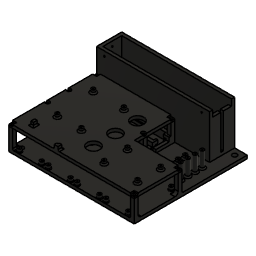
electronics_baseplate (Autodesk Fusion 360 design; units mm, degrees)
Autodesk Fusion 360 part; units mm, degrees
(part 1 of 2)
sketch "Sketch1" plane through (0, 0, 0) normal (0, 1, 0) x (1, 0, 0)
  line L0 (0, 0) -> (200, 0)
  line L1 (200, 0) -> (200, 180)
  line L2 (200, 180) -> (0, 180)
  line L3 (0, 180) -> (0, 0)
  dimension "d3_1" = 200
  dimension "d4_1" = 180
  constraint horizontal L0
  constraint vertical L1
  constraint horizontal L2
  constraint vertical L3
  constraint coincident L0.start L3.end
  measures "d3_1" distance of L0.start L0.end
  measures "d4_1" distance of L0.start L2.end
extrude "Extrude1" add sketch "Sketch1" along normal blind 5 makes body 1
sketch "Sketch3" plane through (0, 0, 0) normal (0, -1, 0) x (1, 0, 0)
  line L0 (0, 0) -> (0, -180)
  line L1 (0, -180) -> (200, -180)
  line L2 (200, -180) -> (200, 0)
  line L3 (200, 0) -> (0, 0)
  line L4 (10, -170) -> (190, -170)
  line L5 (190, -170) -> (190, -10)
  line L6 (190, -10) -> (10, -10)
  line L7 (10, -10) -> (10, -170)
  circle A0 centre (10, -10) radius 2
  circle A1 centre (190, -10) radius 2
  circle A2 centre (10, -170) radius 2
  circle A3 centre (190, -170) radius 2
  dimension "d13_1" = 4
  dimension "d14_1" = 4
  dimension "d15_2" = 4
  dimension "d16" = 4
  constraint coincident L6.end L7.start
  constraint coincident L5.end L6.start
  constraint coincident L4.start L7.end
  constraint coincident L4.end L5.start
  measures "d13_1" diameter of A0
  measures "d14_1" diameter of A1
  measures "d15_2" diameter of A2
  measures "d16" diameter of A3
extrude "Extrude2" cut sketch "Sketch3" against normal up to surface (5 mm away) contours L4 L7 A2 | L4 L7 A2 | L4 L5 A3 | L4 L5 A3 | L6 L7 A0 | L6 L7 A0 | L5 L6 A1 | L5 L6 A1 bodies 1
chamfer "Chamfer1" distance 1.75 distance2 5 4 edges at (8.1353, 5, -170.7232) (188.1353, 5, -170.7232) (8.1353, 5, -10.7232) (188.1353, 5, -10.7232) measured on face at (70.4714, 5, -116.1953) measured on face at (70.4714, 5, -116.1953) measured on face at (70.4714, 5, -116.1953) measured on face at (70.4714, 5, -116.1953) on bodies 1
sketch "Sketch4" plane through (0, 5, 0) normal (0, 1, 0) x (-1, 0, 0)
  circle A0 centre (-10, -10) radius 3.75
  circle A1 centre (-10, -170) radius 3.75
  line L0 (0, -180) -> (0, 0)
  line L1 (0, 0) -> (-200, 0)
  line L2 (-200, 0) -> (-200, -180)
  line L3 (-200, -180) -> (0, -180)
  circle A2 centre (-190, -170) radius 3.75
  circle A3 centre (-190, -10) radius 3.75
  line L4 (0, -180) -> (-180, -180)
  line L5 (-180, -180) -> (-180, -140)
  line L6 (-180, -140) -> (0, -140)
  line L7 (0, -140) -> (0, -180)
  line L8 (-5, -175) -> (-175, -175)
  line L9 (-175, -175) -> (-175, -145)
  line L10 (-175, -145) -> (-5, -145)
  line L11 (-5, -145) -> (-5, -175)
  dimension "d25_1" = 180
  dimension "d26_2" = 40
  dimension "d27_2" = 5
  constraint horizontal L4
  constraint vertical L5
  constraint horizontal L6
  constraint vertical L7
  constraint coincident L0.start L3.end
  measures "d25_1" distance of L0.start L4.end
  measures "d26_2" distance of L0.start L6.end
extrude "Extrude3" add sketch "Sketch4" along normal blind 70 contours L0 L3 L4 L5 L6 L7 bodies 1
sketch "Sketch5" plane through (0, 75, 0) normal (0, 1, 0) x (-1, 0, 0)
  line L0 (-175, -145) -> (-5, -145)
  line L1 (-5, -145) -> (-5, -175)
  line L2 (-5, -175) -> (-175, -175)
  line L3 (-175, -175) -> (-175, -145)
  line L4 (0, -140) -> (-180, -140)
  line L5 (-180, -140) -> (-180, -180)
  line L6 (-180, -180) -> (0, -180)
  line L7 (0, -180) -> (0, -140)
  line L8 (-180, -180) -> (-175, -180)
  line L9 (-175, -180) -> (-175, -175)
  line L10 (-175, -175) -> (-180, -175)
  line L11 (-180, -175) -> (-180, -180)
  line L12 (-175, -145) -> (-180, -145)
  line L13 (-180, -145) -> (-180, -140)
  line L14 (-180, -140) -> (-175, -140)
  line L15 (-175, -140) -> (-175, -145)
  constraint horizontal L8
  constraint vertical L9
  constraint horizontal L10
  constraint vertical L11
  constraint coincident L2.end L3.start
  constraint coincident L5.end L6.start
  constraint horizontal L12
  constraint vertical L13
  constraint horizontal L14
  constraint vertical L15
  constraint coincident L4.end L5.start
  constraint coincident L0.start L3.end
extrude "Extrude4" cut sketch "Sketch5" against normal blind 10 contours L3 L5 L10 L12 bodies 1
sketch "Sketch6" plane through (0, 65, 0) normal (0, 1, 0) x (-1, 0, 0)
  line L0 (-175, -175) -> (-175, -145)
  line L1 (-175, -145) -> (-180, -145)
  line L2 (-180, -145) -> (-180, -175)
  line L3 (-180, -175) -> (-175, -175)
  line L4 (-175, -160) -> (-180, -160)
  line L5 (-180, -162) -> (-175, -162)
  line L6 (-175, -162) -> (-175, -158)
  line L7 (-175, -158) -> (-180, -158)
  line L8 (-180, -158) -> (-180, -162)
  line L9 (-180, -162) -> (-175, -158) construction
  line L10 (-175, -162) -> (-180, -158) construction
  point P0 (-177.5, -160)
  dimension "d34_2" = 5
  dimension "d35_2" = 4
  constraint midpoint L0 L4.start
  constraint midpoint L2 L4.end
  constraint horizontal L5
  constraint perpendicular L5 L6
  constraint parallel L5 L7
  constraint parallel L6 L8
  constraint coincident L9 P0
  constraint coincident L10 P0
  constraint midpoint L4 P0
  measures "d34_2" distance of L6.end L7.end
  measures "d35_2" distance of L5.end L6.end
extrude "Extrude5" cut sketch "Sketch6" against normal blind 55 contours L0 L2 L4 L5 L6 L8 | L0 L2 L4 L6 L7 L8 bodies 1
sketch "Sketch7" plane through (0, 5, 0) normal (0, 1, 0) x (-1, 0, 0)
  circle A0 centre (-190, -10) radius 3.75
  circle A1 centre (-190, -170) radius 3.75
  line L0 (-180, -180) -> (-180, -140)
  line L1 (-180, -140) -> (0, -140)
  line L2 (0, -140) -> (0, 0)
  line L3 (0, 0) -> (-200, 0)
  line L4 (-200, 0) -> (-200, -180)
  line L5 (-200, -180) -> (-180, -180)
  circle A2 centre (-10, -10) radius 3.75
  line L6 (-100, 0) -> (-100, -140)
  line L7 (-100, 0) -> (-98.5, 0)
  line L8 (-98.5, 0) -> (-98.5, -76)
  line L9 (-98.5, -76) -> (-100, -76)
  line L10 (-100, -76) -> (-100, 0)
  line L11 (-98.5, 0) -> (-55.5, 0)
  line L12 (-55.5, 0) -> (-55.5, -76)
  line L13 (-55.5, -76) -> (-98.5, -76)
  line L14 (-98.5, -76) -> (-98.5, 0)
  line L15 (-55.5, 0) -> (-52.5, 0)
  line L16 (-52.5, 0) -> (-52.5, -76)
  line L17 (-52.5, -76) -> (-55.5, -76)
  line L18 (-55.5, -76) -> (-55.5, 0)
  line L19 (-52.5, 0) -> (-9.5, 0)
  line L20 (-9.5, 0) -> (-9.5, -76)
  line L21 (-9.5, -76) -> (-52.5, -76)
  line L22 (-52.5, -76) -> (-52.5, 0)
  line L23 (-48.75, -3.75) -> (-13.25, -3.75)
  line L24 (-13.25, -3.75) -> (-13.25, -72.25)
  line L25 (-13.25, -72.25) -> (-48.75, -72.25)
  line L26 (-48.75, -72.25) -> (-48.75, -3.75)
  line L27 (-59.25, -3.75) -> (-59.25, -72.25)
  line L28 (-59.25, -72.25) -> (-94.75, -72.25)
  line L29 (-94.75, -72.25) -> (-94.75, -3.75)
  line L30 (-94.75, -3.75) -> (-59.25, -3.75)
  circle A3 centre (-13.25, -3.75) radius 3
  circle A4 centre (-13.25, -72.25) radius 3
  circle A5 centre (-48.75, -72.25) radius 3
  circle A6 centre (-59.25, -72.25) radius 3
  circle A7 centre (-94.75, -72.25) radius 3
  circle A8 centre (-59.25, -3.75) radius 3
  circle A9 centre (-94.75, -3.75) radius 3
  line L31 (-100, -76) -> (-100, 0)
  line L32 (-101.5, -76) -> (-101.5, 0)
  line L33 (-147.5, -76) -> (-144.5, -76)
  circle A10 centre (-140.75, -3.75) radius 3
  line L34 (-101.5, 0) -> (-101.5, -76)
  line L35 (-147.5, 0) -> (-147.5, -76)
  line L36 (-190.5, 0) -> (-190.5, -76)
  line L37 (-144.5, 0) -> (-147.5, 0)
  line L38 (-147.5, -76) -> (-147.5, 0)
  line L39 (-144.5, 0) -> (-144.5, -76)
  line L40 (-140.75, -72.25) -> (-105.25, -72.25)
  line L41 (-105.25, -72.25) -> (-105.25, -3.75)
  line L42 (-140.75, -3.75) -> (-140.75, -72.25)
  line L43 (-101.5, 0) -> (-144.5, 0)
  line L44 (-147.5, 0) -> (-190.5, 0)
  circle A11 centre (-186.75, -72.25) radius 3
  circle A12 centre (-151.25, -72.25) radius 3
  line L45 (-151.25, -72.25) -> (-151.25, -3.75)
  circle A13 centre (-186.75, -3.75) radius 3
  line L46 (-101.5, -76) -> (-100, -76)
  line L47 (-144.5, -76) -> (-101.5, -76)
  line L48 (-100, 0) -> (-101.5, 0)
  line L49 (-105.25, -3.75) -> (-140.75, -3.75)
  circle A14 centre (-105.25, -3.75) radius 3
  circle A15 centre (-105.25, -72.25) radius 3
  line L50 (-144.5, -76) -> (-144.5, 0)
  line L51 (-186.75, -72.25) -> (-151.25, -72.25)
  circle A16 centre (-140.75, -72.25) radius 3
  line L52 (-186.75, -3.75) -> (-186.75, -72.25)
  line L53 (-190.5, -76) -> (-147.5, -76)
  line L54 (-151.25, -3.75) -> (-186.75, -3.75)
  circle A17 centre (-48.75, -3.75) radius 3
  circle A18 centre (-151.25, -3.75) radius 3
  point P0 (-190, -10)
  dimension "d46_2" = 1.5
  dimension "d47_2" = 76
  dimension "d48_2" = 43
  dimension "d49_2" = 76
  dimension "d50_2" = 3
  dimension "d51_2" = 76
  dimension "d52_2" = 43
  dimension "d53_2" = 76
  dimension "d54_2" = 3.75
  dimension "d55_2" = 3.75
  dimension "d56_2" = 6
  dimension "d57_2" = 6
  dimension "d58_2" = 6
  dimension "d59_2" = 6
  dimension "d60_2" = 6
  dimension "d61_2" = 6
  dimension "d62_2" = 6
  dimension "d63_2" = 6
  constraint midpoint L3 L6.start
  constraint coincident L1 L6.end
  constraint perpendicular L1 L6
  constraint horizontal L7
  constraint vertical L8
  constraint horizontal L9
  constraint vertical L10
  constraint horizontal L11
  constraint vertical L12
  constraint horizontal L13
  constraint vertical L14
  constraint horizontal L15
  constraint vertical L16
  constraint horizontal L17
  constraint vertical L18
  constraint horizontal L19
  constraint vertical L20
  constraint horizontal L21
  constraint vertical L22
  constraint coincident L23.end L24.start
  constraint coincident L24.end L25.start
  constraint coincident L25.end L26.start
  constraint coincident L27.end L28.start
  constraint coincident L28.end L29.start
  constraint coincident L27.start L30.end
  constraint coincident L29.end L30.start
  constraint symmetric A2.centre L6 P0
  constraint symmetric L7.start L6 L10.end
  constraint symmetric L6 L7.end L32.end
  constraint symmetric L6 L8.end L32.start
  constraint symmetric L6 L9.end L10.start
  constraint symmetric L6 L11.end L37.start
  constraint symmetric L6 L12.end L33.end
  constraint symmetric L6 L15.end L35.start
  constraint symmetric L6 L16.end L33.start
  constraint symmetric L6 L19.end L36.start
  constraint symmetric L6 L20.end L36.end
  constraint symmetric L6 L23.start L45.end
  constraint symmetric L6 L23.end A13.centre
  constraint symmetric L6 L24.end A11.centre
  constraint symmetric L6 L25.end A12.centre
  constraint symmetric L6 L27.start A10.centre
  constraint symmetric L6 L27.end L40.start
  constraint symmetric L6 L28.end L40.end
  constraint symmetric L6 L29.end L41.end
  constraint symmetric L6 A3 A13
  constraint symmetric L6 A4 A11
  constraint symmetric L6 A5 A12
  constraint symmetric L6 A6 A16
  constraint symmetric L6 A7 A15
  constraint symmetric L6 A8 A10
  constraint symmetric L6 A9 A14
  constraint coincident L23.start L26.end
  constraint symmetric L6 A17 A18
  measures "d46_2" distance of L6.start L7.end
  measures "d47_2" distance of L6.start L9.end
  measures "d48_2" distance of L7.end L11.end
  measures "d49_2" distance of L7.end L8.end
  measures "d50_2" distance of L11.end L15.end
  measures "d51_2" distance of L11.end L12.end
  measures "d52_2" distance of L15.end L19.end
  measures "d53_2" distance of L15.end L16.end
  measures "d56_2" diameter of A3
  measures "d57_2" diameter of A4
  measures "d58_2" diameter of A5
  measures "d59_2" diameter of A6
  measures "d60_2" diameter of A7
  measures "d61_2" diameter of A8
  measures "d62_2" diameter of A9
  measures "d63_2" diameter of A17
extrude "Extrude6" add sketch "Sketch7" along normal blind 5 contours A13 L52 L54 | A13 L52 L54 | A11 L51 L52 | A11 L51 L52 | L45 L54 A18 | L45 L54 A18 | A12 L45 L51 | A12 L45 L51 | L23 L24 A3 | L23 L24 A3 | L24 L25 A4 | L24 L25 A4 | L23 L26 A17 | L23 L26 A17 | L25 L26 A5 | L25 L26 A5 | L27 L30 A8 | L27 L30 A8 | L27 L28 A6 | L27 L28 A6 | L29 L30 A9 | L29 L30 A9 | L28 L29 A7 | L28 L29 A7 | A10 L42 L49 | A10 L42 L49 | L41 L49 A14 | L41 L49 A14 | L40 L42 A16 | L40 L42 A16 | L40 L41 A15 | L40 L41 A15 bodies 1
fillet "Fillet1" radius 1 16 edges at (16.047, 5, -71.1652) (51.547, 5, -71.1652) (62.047, 5, -71.1652) (16.047, 5, -2.6652) (51.547, 5, -2.6652) (62.047, 5, -2.6652) (97.547, 5, -71.1652) (108.047, 5, -71.1652) (97.547, 5, -2.6652) (108.047, 5, -2.6652) (143.547, 5, -71.1652) (154.047, 5, -71.1652) (143.547, 5, -2.6652) (154.047, 5, -2.6652) (189.547, 5, -71.1652) (189.547, 5, -2.6652) on bodies 1
sketch "Sketch8" plane through (0, 5, 0) normal (0, 1, 0) x (-1, 0, 0)
  arc A0 (-188.1419, 0) -> (-189.8707, -6.2522) centre (-186.75, -3.75) ccw
  line L0 (-188.1419, 0) -> (-200, 0)
  line L1 (-200, 0) -> (-200, -180)
  line L2 (-200, -180) -> (-180, -180)
  line L3 (-180, -180) -> (-180, -140)
  line L4 (-180, -140) -> (0, -140)
  line L5 (0, -140) -> (0, 0)
  line L6 (0, 0) -> (-11.8581, 0)
  arc A1 (-10.1293, -6.2522) -> (-11.8581, 0) centre (-13.25, -3.75) ccw
  arc A2 (-12.9938, -7.7418) -> (-10.1293, -6.2522) centre (-10, -10) ccw
  arc A3 (-14.6419, 0) -> (-12.9938, -7.7418) centre (-13.25, -3.75) ccw
  line L7 (-14.6419, 0) -> (-47.3581, 0)
  arc A4 (-50.1419, 0) -> (-47.3581, 0) centre (-48.75, -3.75) ccw
  line L8 (-50.1419, 0) -> (-57.8581, 0)
  arc A5 (-60.6419, 0) -> (-57.8581, 0) centre (-59.25, -3.75) ccw
  line L9 (-60.6419, 0) -> (-93.3581, 0)
  arc A6 (-96.1419, 0) -> (-93.3581, 0) centre (-94.75, -3.75) ccw
  line L10 (-96.1419, 0) -> (-103.8581, 0)
  arc A7 (-106.6419, 0) -> (-103.8581, 0) centre (-105.25, -3.75) ccw
  line L11 (-106.6419, 0) -> (-139.3581, 0)
  arc A8 (-142.1419, 0) -> (-139.3581, 0) centre (-140.75, -3.75) ccw
  line L12 (-142.1419, 0) -> (-149.8581, 0)
  arc A9 (-152.6419, 0) -> (-149.8581, 0) centre (-151.25, -3.75) ccw
  line L13 (-152.6419, 0) -> (-185.3581, 0)
  arc A10 (-187.0062, -7.7418) -> (-185.3581, 0) centre (-186.75, -3.75) ccw
  arc A11 (-189.8707, -6.2522) -> (-187.0062, -7.7418) centre (-190, -10) ccw
  circle A12 centre (-151.25, -72.25) radius 4
  circle A13 centre (-105.25, -72.25) radius 4
  circle A14 centre (-59.25, -72.25) radius 4
  circle A15 centre (-13.25, -72.25) radius 4
  circle A16 centre (-190, -170) radius 3.75
  circle A17 centre (-48.75, -72.25) radius 4
  circle A18 centre (-94.75, -72.25) radius 4
  circle A19 centre (-140.75, -72.25) radius 4
  circle A20 centre (-186.75, -72.25) radius 4
  line L14 (0, -140) -> (-55.5, -140)
  line L15 (-55.5, -140) -> (-55.5, -110)
  line L16 (-55.5, -110) -> (0, -110)
  line L17 (0, -110) -> (0, -140)
  line L18 (-55.5, -140) -> (-124.5, -140)
  line L19 (-124.5, -140) -> (-124.5, -110)
  line L20 (-124.5, -110) -> (-55.5, -110)
  line L21 (-55.5, -110) -> (-55.5, -140)
  line L22 (-60.5, -135) -> (-119.5, -135)
  line L23 (-119.5, -135) -> (-119.5, -115)
  line L24 (-119.5, -115) -> (-60.5, -115)
  line L25 (-60.5, -115) -> (-60.5, -135)
  line L26 (-60.5, -135) -> (-61.5, -135)
  line L27 (-61.5, -135) -> (-61.5, -115)
  line L28 (-61.5, -115) -> (-60.5, -115)
  line L29 (-60.5, -115) -> (-60.5, -135)
  line L30 (-60.5, -135) -> (-85.5, -135)
  line L31 (-85.5, -135) -> (-85.5, -134)
  line L32 (-85.5, -134) -> (-60.5, -134)
  line L33 (-60.5, -134) -> (-60.5, -135)
  line L34 (-119.5, -135) -> (-115.5, -135)
  line L35 (-115.5, -135) -> (-115.5, -131)
  line L36 (-115.5, -131) -> (-119.5, -131)
  line L37 (-119.5, -131) -> (-119.5, -135)
  line L38 (-119.5, -115) -> (-115.5, -115)
  line L39 (-115.5, -115) -> (-115.5, -119)
  line L40 (-115.5, -119) -> (-119.5, -119)
  line L41 (-119.5, -119) -> (-119.5, -115)
  line L42 (-119.5, -115) -> (-119.5, -110)
  line L43 (-119.5, -119) -> (-124.5, -119)
  line L44 (-119.5, -131) -> (-124.5, -131)
  line L45 (-60.5, -115) -> (-60.5, -110)
  dimension "d78_1" = 55.5
  dimension "d79_1" = 30
  dimension "d81_1" = 69
  dimension "d82_1" = 30
  dimension "d83_1" = 5
  dimension "d84_1" = 1
  dimension "d85_1" = 25
  dimension "d86_1" = 1
  dimension "d87_1" = 4
  dimension "d88_1" = 4
  dimension "d89_2" = 4
  dimension "d90_2" = 4
  constraint horizontal L14
  constraint vertical L15
  constraint horizontal L16
  constraint vertical L17
  constraint coincident L4.end L5.start
  constraint horizontal L18
  constraint vertical L19
  constraint horizontal L20
  constraint vertical L21
  constraint horizontal L26
  constraint vertical L27
  constraint horizontal L28
  constraint vertical L29
  constraint horizontal L30
  constraint vertical L31
  constraint horizontal L32
  constraint vertical L33
  constraint collinear L24 L28
  constraint horizontal L34
  constraint vertical L35
  constraint horizontal L36
  constraint vertical L37
  constraint horizontal L38
  constraint vertical L39
  constraint horizontal L40
  constraint vertical L41
  constraint coincident L20 L42.end
  constraint perpendicular L20 L42
  constraint coincident L19 L43.end
  constraint perpendicular L19 L43
  constraint coincident L19 L44.end
  constraint perpendicular L19 L44
  constraint coincident L20 L45.end
  constraint perpendicular L20 L45
  measures "d78_1" distance of L4.end L14.end
  measures "d79_1" distance of L4.end L16.end
  measures "d81_1" distance of L14.end L18.end
  measures "d82_1" distance of L14.end L15.end
  measures "d84_1" distance of L22.start L26.end
  measures "d85_1" distance of L22.start L30.end
  measures "d86_1" distance of L22.start L32.end
  measures "d87_1" distance of L22.end L34.end
  measures "d88_1" distance of L22.end L36.end
  measures "d89_2" distance of L23.end L38.end
  measures "d90_2" distance of L23.end L40.end
extrude "Extrude7" add sketch "Sketch8" along normal blind 11.5 contours L4 L15 L18 L19 L20 L21 L22 L23 L25 L26 L29 L30 L33 L34 L37 L44 L45 | L19 L20 L23 L41 L42 L43 | L22 L23 L34 L35 L36 L37 | L24 L25 L27 L28 L29 L32 | L22 L25 L26 L27 L29 L30 L32 L33 | L22 L27 L30 L31 L32 bodies 1
extrude "Extrude8" add sketch "Sketch8" along normal blind 5 contours L19 L23 L43 L44 | L20 L24 L28 L38 L42 L45 | L23 L24 L38 L39 L40 L41 bodies 1
sketch "Sketch9" plane through (0, 0, -110) normal (0, 0, 1) x (1, 0, 0)
  line L0 (55.5, 5) -> (124.5, 5)
  line L1 (124.5, 5) -> (124.5, 16.5)
  line L2 (124.5, 16.5) -> (119.5, 16.5)
  line L3 (119.5, 16.5) -> (119.5, 10)
  line L4 (119.5, 10) -> (60.5, 10)
  line L5 (60.5, 10) -> (60.5, 16.5)
  line L6 (60.5, 16.5) -> (55.5, 16.5)
  line L7 (55.5, 16.5) -> (55.5, 5)
  line L8 (60.5, 10) -> (119.5, 10)
  line L9 (119.5, 10) -> (119.5, 12)
  line L10 (119.5, 12) -> (60.5, 12)
  line L11 (60.5, 12) -> (60.5, 10)
  dimension "d95_1" = 2
  constraint horizontal L8
  constraint vertical L9
  constraint horizontal L10
  constraint vertical L11
  constraint coincident L3 L9.end
  constraint coincident L4.end L5.start
  measures "d95_1" distance of L4.end L10.end
extrude "Extrude9" cut sketch "Sketch9" against normal up to surface (25 mm away) contours L3 L4 L5 L8 L9 L10 L11 bodies 1
sketch "Sketch14" plane through (0, 0, -110) normal (0, 0, 1) x (1, 0, 0)
  line L0 (55.5, 5) -> (124.5, 5)
  line L1 (124.5, 5) -> (124.5, 16.5)
  line L2 (124.5, 16.5) -> (119.5, 16.5)
  line L3 (119.5, 16.5) -> (119.5, 10)
  line L4 (119.5, 10) -> (60.5, 10)
  line L5 (60.5, 10) -> (60.5, 16.5)
  line L6 (60.5, 16.5) -> (55.5, 16.5)
  line L7 (55.5, 16.5) -> (55.5, 5)
  line L8 (60.5, 5) -> (119.5, 5)
  line L9 (119.5, 5) -> (119.5, 10)
  line L10 (119.5, 10) -> (60.5, 10)
  line L11 (60.5, 10) -> (60.5, 5)
  line L12 (60.5, 10) -> (64.5, 10)
  line L13 (64.5, 10) -> (64.5, 5)
  line L14 (64.5, 5) -> (60.5, 5)
  line L15 (60.5, 5) -> (60.5, 10)
  line L16 (119.5, 10) -> (115.5, 10)
  line L17 (115.5, 10) -> (115.5, 5)
  line L18 (115.5, 5) -> (119.5, 5)
  line L19 (119.5, 5) -> (119.5, 10)
  line L20 (64.5, 10) -> (68.5, 10)
  line L21 (68.5, 10) -> (68.5, 7)
  line L22 (68.5, 7) -> (64.5, 7)
  line L23 (64.5, 7) -> (64.5, 10)
  line L24 (115.5, 10) -> (111.5, 10)
  line L25 (111.5, 10) -> (111.5, 7)
  line L26 (111.5, 7) -> (115.5, 7)
  line L27 (115.5, 7) -> (115.5, 10)
  line L28 (68.5, 7) -> (111.5, 7)
  line L29 (90, 10) -> (90, 7)
  line L30 (115.5, 7) -> (119.5, 7)
  line L31 (88, 10) -> (92, 10)
  line L32 (92, 10) -> (92, 7)
  line L33 (92, 7) -> (88, 7)
  line L34 (88, 7) -> (88, 10)
  line L35 (88, 10) -> (92, 7) construction
  line L36 (92, 10) -> (88, 7) construction
  point P0 (90, 8.5)
  dimension "d106_1" = 4
  dimension "d107_1" = 4
  dimension "d108_1" = 4
  dimension "d109" = 3
  dimension "d110" = 4
  dimension "d111_1" = 3
  dimension "d112_1" = 4
  constraint horizontal L8
  constraint vertical L9
  constraint horizontal L10
  constraint vertical L11
  constraint coincident L3.end L4.start
  constraint coincident L0 L8.start
  constraint collinear L5 L11
  constraint horizontal L12
  constraint vertical L13
  constraint horizontal L14
  constraint vertical L15
  constraint horizontal L16
  constraint vertical L17
  constraint horizontal L18
  constraint vertical L19
  constraint collinear L8 L14
  constraint collinear L8 L18
  constraint horizontal L20
  constraint vertical L21
  constraint horizontal L22
  constraint vertical L23
  constraint horizontal L24
  constraint vertical L25
  constraint horizontal L26
  constraint vertical L27
  constraint midpoint L10 L29.start
  constraint midpoint L28 L29.end
  constraint coincident L9 L30.end
  constraint perpendicular L9 L30
  constraint horizontal L31
  constraint perpendicular L31 L32
  constraint parallel L31 L33
  constraint parallel L32 L34
  constraint coincident L35 P0
  constraint coincident L36 P0
  constraint midpoint L29 P0
  constraint collinear L10 L31
  measures "d106_1" distance of L4.end L12.end
  measures "d107_1" distance of L3.end L16.end
  measures "d108_1" distance of L12.end L20.end
  measures "d109" distance of L12.end L22.end
  measures "d110" distance of L16.end L24.end
  measures "d111_1" distance of L16.end L26.end
  measures "d112_1" distance of L32.end L33.end
extrude "Extrude11" cut sketch "Sketch14" against normal up to surface (5 mm away) contours L4 L10 L13 L20 L21 L22 L23 | L4 L10 L17 L24 L25 L26 L27 | L4 L10 L28 L29 L31 L33 L34 | L4 L10 L28 L29 L31 L32 L33 bodies 1
extrude "Extrude12" cut sketch "Sketch14" against normal up to surface (9 mm away) contours L4 L9 L10 L16 L17 L19 L27 L30 bodies 1
sketch "Sketch15" plane through (0, 5, 0) normal (0, 1, 0) x (-1, 0, 0)
  line L0 (-124.5, -110) -> (-55.5, -110)
  line L1 (-55.5, -110) -> (-55.5, -140)
  line L2 (-55.5, -140) -> (0, -140)
  line L3 (0, -140) -> (0, 0)
  line L4 (0, 0) -> (-11.8581, 0)
  arc A0 (-10.1293, -6.2522) -> (-11.8581, 0) centre (-13.25, -3.75) ccw
  arc A1 (-12.9938, -7.7418) -> (-10.1293, -6.2522) centre (-10, -10) ccw
  arc A2 (-14.6419, 0) -> (-12.9938, -7.7418) centre (-13.25, -3.75) ccw
  line L5 (-14.6419, 0) -> (-47.3581, 0)
  arc A3 (-50.1419, 0) -> (-47.3581, 0) centre (-48.75, -3.75) ccw
  line L6 (-50.1419, 0) -> (-57.8581, 0)
  arc A4 (-60.6419, 0) -> (-57.8581, 0) centre (-59.25, -3.75) ccw
  line L7 (-60.6419, 0) -> (-93.3581, 0)
  arc A5 (-96.1419, 0) -> (-93.3581, 0) centre (-94.75, -3.75) ccw
  line L8 (-96.1419, 0) -> (-103.8581, 0)
  arc A6 (-106.6419, 0) -> (-103.8581, 0) centre (-105.25, -3.75) ccw
  line L9 (-106.6419, 0) -> (-139.3581, 0)
  arc A7 (-142.1419, 0) -> (-139.3581, 0) centre (-140.75, -3.75) ccw
  line L10 (-142.1419, 0) -> (-149.8581, 0)
  arc A8 (-152.6419, 0) -> (-149.8581, 0) centre (-151.25, -3.75) ccw
  line L11 (-152.6419, 0) -> (-185.3581, 0)
  arc A9 (-187.0062, -7.7418) -> (-185.3581, 0) centre (-186.75, -3.75) ccw
  arc A10 (-189.8707, -6.2522) -> (-187.0062, -7.7418) centre (-190, -10) ccw
  arc A11 (-188.1419, 0) -> (-189.8707, -6.2522) centre (-186.75, -3.75) ccw
  line L12 (-188.1419, 0) -> (-200, 0)
  line L13 (-200, 0) -> (-200, -180)
  line L14 (-200, -180) -> (-180, -180)
  line L15 (-180, -180) -> (-180, -140)
  line L16 (-180, -140) -> (-124.5, -140)
  line L17 (-124.5, -140) -> (-124.5, -110)
  circle A12 centre (-151.25, -72.25) radius 4
  circle A13 centre (-105.25, -72.25) radius 4
  circle A14 centre (-59.25, -72.25) radius 4
  circle A15 centre (-13.25, -72.25) radius 4
  circle A16 centre (-190, -170) radius 3.75
  circle A17 centre (-48.75, -72.25) radius 4
  circle A18 centre (-94.75, -72.25) radius 4
  circle A19 centre (-140.75, -72.25) radius 4
  circle A20 centre (-186.75, -72.25) radius 4
  line L18 (-200, 0) -> (0, 0)
  line L19 (0, 0) -> (0, -76)
  line L20 (0, -76) -> (-200, -76)
  line L21 (-200, -76) -> (-200, 0)
  line L22 (0, -140) -> (-200, -140)
  line L23 (-195, 0) -> (-195, -180)
  line L24 (0, -132.5) -> (-200, -132.5)
  line L25 (-195, -132.5) -> (-168, -132.5)
  line L26 (-168, -132.5) -> (-168, -126.75)
  line L27 (-168, -126.75) -> (-195, -126.75)
  line L28 (-195, -126.75) -> (-195, -132.5)
  line L29 (-195, -126.75) -> (-168, -126.75)
  line L30 (-168, -126.75) -> (-168, -115.25)
  line L31 (-168, -115.25) -> (-195, -115.25)
  line L32 (-195, -115.25) -> (-195, -126.75)
  line L33 (-168, -115.25) -> (-168, -126.75)
  line L34 (-141, -126.75) -> (-168, -126.75)
  line L35 (-141, -115.25) -> (-168, -115.25)
  line L36 (-168, -126.75) -> (-141, -126.75)
  line L37 (-141, -126.75) -> (-141, -115.25)
  line L38 (-195, -103.75) -> (-195, -115.25)
  line L39 (-168, -115.25) -> (-195, -115.25)
  line L40 (-168, -103.75) -> (-195, -103.75)
  line L41 (-195, -115.25) -> (-168, -115.25)
  line L42 (-168, -115.25) -> (-168, -103.75)
  line L43 (-168, -103.75) -> (-168, -115.25)
  line L44 (-141, -115.25) -> (-168, -115.25)
  line L45 (-141, -103.75) -> (-168, -103.75)
  line L46 (-168, -115.25) -> (-141, -115.25)
  line L47 (-141, -115.25) -> (-141, -103.75)
  line L48 (-195, -92.25) -> (-195, -103.75)
  line L49 (-168, -103.75) -> (-195, -103.75)
  line L50 (-168, -92.25) -> (-195, -92.25)
  line L51 (-195, -103.75) -> (-168, -103.75)
  line L52 (-168, -103.75) -> (-168, -92.25)
  line L53 (-168, -92.25) -> (-168, -103.75)
  line L54 (-141, -103.75) -> (-168, -103.75)
  line L55 (-141, -92.25) -> (-168, -92.25)
  line L56 (-168, -103.75) -> (-141, -103.75)
  line L57 (-141, -103.75) -> (-141, -92.25)
  line L58 (-195, -80.75) -> (-195, -92.25)
  line L59 (-168, -92.25) -> (-195, -92.25)
  line L60 (-168, -80.75) -> (-195, -80.75)
  line L61 (-195, -92.25) -> (-168, -92.25)
  line L62 (-168, -92.25) -> (-168, -80.75)
  line L63 (-168, -80.75) -> (-168, -92.25)
  line L64 (-141, -92.25) -> (-168, -92.25)
  line L65 (-141, -80.75) -> (-168, -80.75)
  line L66 (-168, -92.25) -> (-141, -92.25)
  line L67 (-141, -92.25) -> (-141, -80.75)
  circle A21 centre (-154.5, -126.75) radius 3
  circle A22 centre (-154.5, -115.25) radius 3
  circle A23 centre (-154.5, -103.75) radius 3
  circle A24 centre (-154.5, -92.25) radius 3
  circle A25 centre (-181.5, -126.75) radius 3
  circle A26 centre (-181.5, -115.25) radius 3
  circle A27 centre (-181.5, -103.75) radius 3
  circle A28 centre (-181.5, -92.25) radius 3
  dimension "d121_1" = 76
  dimension "d130_1" = 7.5
  dimension "d131_1" = 27
  dimension "d132_1" = 5.75
  dimension "d133_1" = 27
  dimension "d134_1" = 11.5
  dimension "d137_1" = 27
  dimension "d138_1" = 11.5
  dimension "d140_1" = 6
  dimension "d141_1" = 6
  dimension "d142_1" = 6
  dimension "d143_1" = 6
  dimension "d144_1" = 6
  dimension "d145_1" = 6
  dimension "d146_1" = 6
  dimension "d147_1" = 6
  constraint horizontal L18
  constraint vertical L19
  constraint horizontal L20
  constraint vertical L21
  constraint coincident L12.end L13.start
  constraint collinear L3 L19
  constraint coincident L2.end L3.start
  constraint coincident L13 L22.end
  constraint perpendicular L13 L22
  constraint horizontal L25
  constraint vertical L26
  constraint horizontal L27
  constraint vertical L28
  constraint coincident L24 L25.start
  constraint coincident L23 L25.start
  constraint horizontal L29
  constraint vertical L30
  constraint horizontal L31
  constraint vertical L32
  constraint midpoint L36 A21.centre
  constraint midpoint L44 A22.centre
  constraint midpoint L56 A23.centre
  constraint midpoint L64 A24.centre
  constraint midpoint L29 A25.centre
  constraint midpoint L31 A26.centre
  constraint midpoint L51 A27.centre
  constraint midpoint L59 A28.centre
  measures "d121_1" distance of L12.end L20.end
  measures "d131_1" distance of L25.start L25.end
  measures "d132_1" distance of L25.start L27.end
  measures "d133_1" distance of L27.end L26.end
  measures "d134_1" distance of L27.end L31.end
  measures "d140_1" diameter of A21
  measures "d141_1" diameter of A22
  measures "d142_1" diameter of A23
  measures "d143_1" diameter of A24
  measures "d144_1" diameter of A25
  measures "d145_1" diameter of A26
  measures "d146_1" diameter of A27
  measures "d147_1" diameter of A28
extrude "Extrude13" add sketch "Sketch15" along normal blind 5 contours L34 L36 A21 | L34 L36 A21 | L35 L44 L46 A22 | L35 L44 L46 A22 | L45 L54 L56 A23 | L45 L54 L56 A23 | L55 L64 L66 A24 | L55 L64 L66 A24 bodies 1
extrude "Extrude14" add sketch "Sketch15" along normal blind 25 contours L27 L29 A25 | L27 L29 A25 | L31 L39 L41 A26 | L31 L39 L41 A26 | L40 L49 L51 A27 | L40 L49 L51 A27 | L50 L59 L61 A28 | L50 L59 L61 A28 bodies 1
fillet "Fillet2" radius 2 8 edges at (157.297, 5, -91.1652) (157.297, 5, -102.6652) (157.297, 5, -114.1652) (157.297, 5, -125.6652) (184.297, 5, -125.6652) (184.297, 5, -114.1652) (184.297, 5, -102.6652) (184.297, 5, -91.1652) on bodies 1
hole "Hole1" at (13.25, 10, -3.75) direction (0, -1, 0) diameter 2.5 end through all bodies 1
hole "Hole2" at (48.75, 10, -3.75) direction (0, -1, 0) diameter 2.5 end through all bodies 1
hole "Hole3" at (59.25, 10, -3.75) direction (0, -1, 0) diameter 2.5 end through all bodies 1
hole "Hole4" at (94.75, 10, -3.75) direction (0, -1, 0) diameter 2.5 end through all bodies 1
hole "Hole5" at (105.25, 10, -3.75) direction (0, -1, 0) diameter 2.5 end through all bodies 1
hole "Hole6" at (140.75, 10, -3.75) direction (0, -1, 0) diameter 2.5 end through all bodies 1
hole "Hole7" at (151.25, 10, -3.75) direction (0, -1, 0) diameter 2.5 end through all bodies 1
hole "Hole8" at (186.75, 10, -3.75) direction (0, -1, 0) diameter 2.5 end through all bodies 1
hole "Hole9" at (13.25, 10, -72.25) direction (0, -1, 0) diameter 2.5 end through all bodies 1
hole "Hole10" at (48.75, 10, -72.25) direction (0, -1, 0) diameter 2.5 end through all bodies 1
hole "Hole11" at (59.25, 10, -72.25) direction (0, -1, 0) diameter 2.5 end through all bodies 1
hole "Hole12" at (94.75, 10, -72.25) direction (0, -1, 0) diameter 2.5 end through all bodies 1
hole "Hole13" at (105.25, 10, -72.25) direction (0, -1, 0) diameter 2.5 end through all bodies 1
hole "Hole14" at (140.75, 10, -72.25) direction (0, -1, 0) diameter 2.5 end through all bodies 1
hole "Hole15" at (151.25, 10, -72.25) direction (0, -1, 0) diameter 2.5 end through all bodies 1
hole "Hole16" at (186.75, 10, -72.25) direction (0, -1, 0) diameter 2.5 end through all bodies 1
hole "Hole17" at (154.5, 10, -92.25) direction (0, -1, 0) diameter 2.5 end through all bodies 1
hole "Hole18" at (154.5, 10, -103.75) direction (0, -1, 0) diameter 2.5 end through all bodies 1
hole "Hole19" at (154.5, 10, -115.25) direction (0, -1, 0) diameter 2.5 end through all bodies 1
hole "Hole20" at (154.5, 10, -126.75) direction (0, -1, 0) diameter 2.5 end through all bodies 1
hole "Hole21" at (181.5, 30, -92.25) direction (0, -1, 0) diameter 2.5 depth 10 tip angle 180 bodies 1
hole "Hole22" at (181.5, 30, -103.75) direction (0, -1, 0) diameter 2.5 depth 10 tip angle 180 bodies 1
hole "Hole23" at (181.5, 30, -115.25) direction (0, -1, 0) diameter 2.5 depth 10 tip angle 180 bodies 1
hole "Hole24" at (181.5, 30, -126.75) direction (0, -1, 0) diameter 2.5 depth 10 tip angle 180 bodies 1
sketch "Sketch19" plane through (0, 5, 0) normal (0, 1, 0) x (-1, 0, 0)
  circle A0 centre (-181.5, -103.75) radius 5
  circle A1 centre (-181.5, -126.75) radius 5
  circle A2 centre (-154.5, -115.25) radius 5
  circle A3 centre (-154.5, -92.25) radius 5
  line L0 (-124.5, -110) -> (-55.5, -110)
  line L1 (-55.5, -110) -> (-55.5, -140)
  line L2 (-55.5, -140) -> (0, -140)
  line L3 (0, -140) -> (0, 0)
  line L4 (0, 0) -> (-11.8581, 0)
  arc A4 (-10.1293, -6.2522) -> (-11.8581, 0) centre (-13.25, -3.75) ccw
  arc A5 (-12.9938, -7.7418) -> (-10.1293, -6.2522) centre (-10, -10) ccw
  arc A6 (-14.6419, 0) -> (-12.9938, -7.7418) centre (-13.25, -3.75) ccw
  line L5 (-14.6419, 0) -> (-47.3581, 0)
  arc A7 (-50.1419, 0) -> (-47.3581, 0) centre (-48.75, -3.75) ccw
  line L6 (-50.1419, 0) -> (-57.8581, 0)
  arc A8 (-60.6419, 0) -> (-57.8581, 0) centre (-59.25, -3.75) ccw
  line L7 (-60.6419, 0) -> (-93.3581, 0)
  arc A9 (-96.1419, 0) -> (-93.3581, 0) centre (-94.75, -3.75) ccw
  line L8 (-96.1419, 0) -> (-103.8581, 0)
  arc A10 (-106.6419, 0) -> (-103.8581, 0) centre (-105.25, -3.75) ccw
  line L9 (-106.6419, 0) -> (-139.3581, 0)
  arc A11 (-142.1419, 0) -> (-139.3581, 0) centre (-140.75, -3.75) ccw
  line L10 (-142.1419, 0) -> (-149.8581, 0)
  arc A12 (-152.6419, 0) -> (-149.8581, 0) centre (-151.25, -3.75) ccw
  line L11 (-152.6419, 0) -> (-185.3581, 0)
  arc A13 (-187.0062, -7.7418) -> (-185.3581, 0) centre (-186.75, -3.75) ccw
  arc A14 (-189.8707, -6.2522) -> (-187.0062, -7.7418) centre (-190, -10) ccw
  arc A15 (-188.1419, 0) -> (-189.8707, -6.2522) centre (-186.75, -3.75) ccw
  line L12 (-188.1419, 0) -> (-200, 0)
  line L13 (-200, 0) -> (-200, -180)
  line L14 (-200, -180) -> (-180, -180)
  line L15 (-180, -180) -> (-180, -140)
  line L16 (-180, -140) -> (-124.5, -140)
  line L17 (-124.5, -140) -> (-124.5, -110)
  circle A16 centre (-151.25, -72.25) radius 4
  circle A17 centre (-105.25, -72.25) radius 4
  circle A18 centre (-59.25, -72.25) radius 4
  circle A19 centre (-13.25, -72.25) radius 4
  circle A20 centre (-190, -170) radius 3.75
  circle A21 centre (-48.75, -72.25) radius 4
  circle A22 centre (-94.75, -72.25) radius 4
  circle A23 centre (-140.75, -72.25) radius 4
  circle A24 centre (-186.75, -72.25) radius 4
  circle A25 centre (-154.5, -103.75) radius 5
  circle A26 centre (-154.5, -126.75) radius 5
  circle A27 centre (-181.5, -115.25) radius 5
  circle A28 centre (-181.5, -92.25) radius 5
  line L18 (0, 0) -> (-6, 0)
  line L19 (-6, 0) -> (-6, -6)
  line L20 (-6, -6) -> (0, -6)
  line L21 (0, -6) -> (0, 0)
  line L22 (0, -140) -> (-6, -140)
  line L23 (-6, -140) -> (-6, -134)
  line L24 (-6, -134) -> (0, -134)
  line L25 (0, -134) -> (0, -140)
  line L26 (-200, 0) -> (-194, 0)
  line L27 (-194, 0) -> (-194, -6)
  line L28 (-194, -6) -> (-200, -6)
  line L29 (-200, -6) -> (-200, 0)
  line L30 (-180, -140) -> (-200, -140)
  line L31 (-200, -140) -> (-194, -140)
  line L32 (-194, -140) -> (-194, -76)
  line L33 (-194, -76) -> (-200, -76)
  line L34 (-200, -76) -> (-200, -140)
  line L35 (-200, -76) -> (-194, -76)
  line L36 (-194, -76) -> (-194, -70)
  line L37 (-194, -70) -> (-200, -70)
  line L38 (-200, -70) -> (-200, -76)
  line L39 (-124.5, -140) -> (-118.5, -140)
  line L40 (-118.5, -140) -> (-118.5, -134)
  line L41 (-118.5, -134) -> (-124.5, -134)
  line L42 (-124.5, -134) -> (-124.5, -140)
  line L43 (-200, -76) -> (0, -76)
  line L44 (-124.5, -110) -> (-124.5, -76)
  line L45 (-124.5, -93) -> (-118.5, -93)
  line L46 (-118.5, -93) -> (-118.5, -96)
  line L47 (-118.5, -96) -> (-124.5, -96)
  line L48 (-124.5, -96) -> (-124.5, -93)
  line L49 (-124.5, -93) -> (-118.5, -93)
  line L50 (-118.5, -93) -> (-118.5, -90)
  line L51 (-118.5, -90) -> (-124.5, -90)
  line L52 (-124.5, -90) -> (-124.5, -93)
  line L53 (0, -140) -> (0, -76)
  line L54 (0, -76) -> (0, 0)
  line L55 (-118.5, -90) -> (0, -90)
  line L56 (0, -90) -> (-6, -90)
  line L57 (-6, -90) -> (-6, -96)
  line L58 (-6, -96) -> (0, -96)
  line L59 (0, -96) -> (0, -90)
  line L60 (-118.5, -62) -> (0, -62)
  line L61 (0, -62) -> (-6, -62)
  line L62 (-6, -62) -> (-6, -56)
  line L63 (-6, -56) -> (0, -56)
  line L64 (0, -56) -> (0, -62)
  dimension "d230_1" = 6
  dimension "d231_1" = 6
  dimension "d232_1" = 6
  dimension "d233_1" = 6
  dimension "d234_1" = 6
  dimension "d235_1" = 6
  dimension "d237_1" = 6
  dimension "d238_1" = 64
  dimension "d239_1" = 6
  dimension "d240_1" = 6
  dimension "d241_1" = 6
  dimension "d242_1" = 6
  dimension "d243_1" = 6
  dimension "d244_1" = 3
  dimension "d245_1" = 6
  dimension "d246_1" = 3
  dimension "d247_1" = 6
  dimension "d248_1" = 6
  dimension "d249_1" = 6
  dimension "d250_1" = 6
  constraint horizontal L18
  constraint vertical L19
  constraint horizontal L20
  constraint vertical L21
  constraint coincident L3.end L4.start
  constraint horizontal L22
  constraint vertical L23
  constraint horizontal L24
  constraint vertical L25
  constraint coincident L2.end L3.start
  constraint horizontal L26
  constraint vertical L27
  constraint horizontal L28
  constraint vertical L29
  constraint coincident L12.end L13.start
  constraint coincident L15.end L16.start
  constraint coincident L13 L30.end
  constraint perpendicular L13 L30
  constraint horizontal L31
  constraint vertical L32
  constraint horizontal L33
  constraint vertical L34
  constraint horizontal L35
  constraint vertical L36
  constraint horizontal L37
  constraint vertical L38
  constraint horizontal L39
  constraint vertical L40
  constraint horizontal L41
  constraint vertical L42
  constraint coincident L16.end L17.start
  constraint coincident L3 L43.end
  constraint perpendicular L3 L43
  constraint coincident L0.start L17.end
  constraint coincident L43 L44.end
  constraint perpendicular L43 L44
  constraint horizontal L45
  constraint vertical L46
  constraint horizontal L47
  constraint vertical L48
  constraint midpoint L44 L45.start
  constraint horizontal L49
  constraint vertical L50
  constraint horizontal L51
  constraint vertical L52
  constraint coincident L53 L55.end
  constraint perpendicular L53 L55
  constraint vertical L57
  constraint perpendicular L56 L57
  constraint horizontal L58
  constraint parallel L57 L59
  constraint symmetric L43 L50.end L60.start
  constraint symmetric L43 L55.end L60.end
  constraint vertical L62
  constraint perpendicular L61 L62
  constraint horizontal L63
  constraint parallel L62 L64
  measures "d230_1" distance of L3.end L18.end
  measures "d231_1" distance of L3.end L20.end
  measures "d232_1" distance of L2.end L22.end
  measures "d233_1" distance of L2.end L24.end
  measures "d234_1" distance of L12.end L26.end
  measures "d235_1" distance of L12.end L28.end
  measures "d237_1" distance of L30.end L31.end
  measures "d238_1" distance of L30.end L33.end
  measures "d239_1" distance of L33.end L32.end
  measures "d240_1" distance of L33.end L37.end
  measures "d241_1" distance of L16.end L39.end
  measures "d242_1" distance of L16.end L41.end
  measures "d243_1" distance of L45.start L45.end
  measures "d244_1" distance of L45.start L47.end
  measures "d245_1" distance of L45.start L45.end
  measures "d246_1" distance of L45.start L51.end
  measures "d247_1" distance of L55.end L56.end
  measures "d248_1" distance of L55.end L58.end
  measures "d249_1" distance of L60.end L61.end
  measures "d250_1" distance of L60.end L63.end
extrude "Extrude15" add sketch "Sketch19" along normal blind 30 contours L17 L39 L40 L41 L42 | L44 L45 L46 L47 L48 L49 | L44 L45 L49 L50 L51 L52 | L2 L3 L22 L23 L24 L25 L53 | L13 L33 L35 L36 L37 L38 L43 | L3 L53 L55 L56 L57 L58 L59 | L12 L13 L26 L27 L28 L29 | L3 L54 L60 L61 L62 L63 L64 | L3 L4 L18 L19 L20 L21 L54 bodies 1
fillet "Fillet3" radius 2 11 edges at (6, 5, -3) (6, 5, -59) (6, 5, -93) (6, 5, -137) (194, 5, -73) (194, 5, -3) (121.5, 5, -90) (124.5, 5, -93) (118.5, 5, -93) (121.5, 5, -96) (197, 5, -76) on bodies 1
fillet "Fillet4" radius 5 8 edges at (4, 5, -134) (4, 5, -90) (4, 5, -56) (196, 5, -70) (4, 5, -6) (4, 5, -62) (196, 5, -6) (4, 5, -96) on bodies 1
hole "Hole25" at (3, 35, -137) direction (0, -1, 0) diameter 2.5 depth 10 tip angle 180 bodies 1
hole "Hole26" at (3, 35, -93) direction (0, -1, 0) diameter 2.5 depth 10 tip angle 180 bodies 1
hole "Hole27" at (3, 35, -59) direction (0, -1, 0) diameter 2.5 depth 10 tip angle 180 bodies 1
hole "Hole28" at (3, 35, -3) direction (0, -1, 0) diameter 2.5 depth 10 tip angle 180 bodies 1
hole "Hole29" at (121.5, 35, -137) direction (0, -1, 0) diameter 2.5 depth 10 tip angle 180 bodies 1
hole "Hole30" at (121.5, 35, -93) direction (0, -1, 0) diameter 2.5 depth 10 tip angle 180 bodies 1
hole "Hole31" at (197, 35, -73) direction (0, -1, 0) diameter 2.5 depth 10 tip angle 180 bodies 1
hole "Hole32" at (197, 35, -3) direction (0, -1, 0) diameter 2.5 depth 10 tip angle 180 bodies 1
sketch "Sketch20" plane through (0, 35, 0) normal (0, 1, 0) x (-1, 0, 0)
  circle A0 centre (-3, -3) radius 1.25
  line L0 (-6, -6) -> (0, -6)
  line L1 (0, -6) -> (0, 0)
  line L2 (0, 0) -> (-6, 0)
  line L3 (-6, 0) -> (-6, -6)
  line L4 (0, 0) -> (-200, 0)
  line L5 (-200, 0) -> (-200, -140)
  line L6 (-200, -140) -> (0, -140)
  line L7 (0, -140) -> (0, 0)
  line L8 (-200, -140) -> (-124.5, -140)
  line L9 (-124.5, -140) -> (-124.5, -76)
  line L10 (-124.5, -76) -> (-200, -76)
  line L11 (-200, -76) -> (-200, -140)
  dimension "d285_1" = 200
  dimension "d286_1" = 140
  dimension "d287_1" = 75.5
  dimension "d288_1" = 64
  constraint horizontal L4
  constraint vertical L5
  constraint horizontal L6
  constraint vertical L7
  constraint coincident L1.end L2.start
  constraint horizontal L8
  constraint vertical L9
  constraint horizontal L10
  constraint vertical L11
  measures "d285_1" distance of L1.end L4.end
  measures "d286_1" distance of L1.end L6.end
  measures "d287_1" distance of L5.end L8.end
  measures "d288_1" distance of L5.end L10.end
extrude "Extrude16" add sketch "Sketch20" along normal blind 5 separate body contours A0 | L0 L1 L2 L3 L4 L7 | L0 L3 L4 L5 L6 L7 L9 L10 makes body 2
sketch "Sketch21" plane through (0, 40, 0) normal (0, 1, 0) x (-1, 0, 0)
  line L0 (-124.5, -140) -> (0, -140)
  line L1 (0, -140) -> (0, 0)
  line L2 (0, 0) -> (-200, 0)
  line L3 (-200, 0) -> (-200, -76)
  line L4 (-200, -76) -> (-124.5, -76)
  line L5 (-124.5, -76) -> (-124.5, -140)
  line L6 (0, -140) -> (-6, -140)
  line L7 (-6, -140) -> (-6, -134)
  line L8 (-6, -134) -> (0, -134)
  line L9 (0, -134) -> (0, -140)
  line L10 (0, 0) -> (-6, 0)
  line L11 (-6, 0) -> (-6, -6)
  line L12 (-6, -6) -> (0, -6)
  line L13 (0, -6) -> (0, 0)
  line L14 (-200, 0) -> (-194, 0)
  line L15 (-194, 0) -> (-194, -6)
  line L16 (-194, -6) -> (-200, -6)
  line L17 (-200, -6) -> (-200, 0)
  line L18 (-200, -76) -> (-194, -76)
  line L19 (-194, -76) -> (-194, -70)
  line L20 (-194, -70) -> (-200, -70)
  line L21 (-200, -70) -> (-200, -76)
  line L22 (-124.5, -140) -> (-118.5, -140)
  line L23 (-118.5, -140) -> (-118.5, -134)
  line L24 (-118.5, -134) -> (-124.5, -134)
  line L25 (-124.5, -134) -> (-124.5, -140)
  line L26 (-124.5, -140) -> (-118.5, -140)
  line L27 (-118.5, -140) -> (-118.5, -110)
  line L28 (-118.5, -110) -> (-124.5, -110)
  line L29 (-124.5, -110) -> (-124.5, -140)
  line L30 (-124.5, -76) -> (0, -76)
  line L31 (-124.5, -110) -> (-124.5, -76)
  line L32 (-124.5, -93) -> (-118.5, -93)
  line L33 (-118.5, -93) -> (-118.5, -96)
  line L34 (-118.5, -96) -> (-124.5, -96)
  line L35 (-124.5, -96) -> (-124.5, -93)
  line L36 (-124.5, -93) -> (-118.5, -93)
  line L37 (-118.5, -93) -> (-118.5, -90)
  line L38 (-118.5, -90) -> (-124.5, -90)
  line L39 (-124.5, -90) -> (-124.5, -93)
  line L40 (-118.5, -90) -> (0, -90)
  line L41 (0, -90) -> (-6, -90)
  line L42 (-6, -90) -> (-6, -96)
  line L43 (-6, -96) -> (0, -96)
  line L44 (0, -96) -> (0, -90)
  line L45 (-118.5, -62) -> (0, -62)
  line L46 (-6, -62) -> (-6, -56)
  line L47 (-6, -56) -> (0, -56)
  line L48 (0, -56) -> (0, -62)
  line L49 (0, -140) -> (-6, -134)
  line L50 (0, -90) -> (-6, -96)
  line L51 (0, -62) -> (-6, -56)
  line L52 (0, 0) -> (-6, -6)
  line L53 (-194, -6) -> (-200, 0)
  line L54 (-194, -76) -> (-200, -70)
  line L55 (-124.5, -140) -> (-118.5, -134)
  circle A0 centre (-3, -3) radius 1.75
  circle A1 centre (-3, -59) radius 1.75
  circle A2 centre (-3, -93) radius 1.75
  circle A3 centre (-3, -137) radius 1.75
  circle A4 centre (-121.5, -137) radius 1.75
  circle A5 centre (-121.5, -93) radius 1.75
  circle A6 centre (-197, -73) radius 1.75
  circle A7 centre (-197, -3) radius 1.75
  dimension "d291_1" = 6
  dimension "d292_1" = 6
  dimension "d293_1" = 6
  dimension "d294_1" = 6
  dimension "d295_1" = 6
  dimension "d296_1" = 6
  dimension "d297_1" = 6
  dimension "d298_1" = 6
  dimension "d299_1" = 6
  dimension "d300_1" = 6
  dimension "d301_1" = 6
  dimension "d302_1" = 30
  dimension "d303_1" = 6
  dimension "d304_1" = 3
  dimension "d305_1" = 6
  dimension "d306_1" = 3
  dimension "d307_1" = 6
  dimension "d308_1" = 6
  dimension "d310_1" = 3.5
  dimension "d311_1" = 3.5
  dimension "d312_1" = 3.5
  dimension "d313_1" = 3.5
  dimension "d314_1" = 3.5
  dimension "d315_1" = 3.5
  dimension "d316_1" = 3.5
  dimension "d317_1" = 3.5
  constraint horizontal L6
  constraint vertical L7
  constraint horizontal L8
  constraint vertical L9
  constraint coincident L0.end L1.start
  constraint horizontal L10
  constraint vertical L11
  constraint horizontal L12
  constraint vertical L13
  constraint coincident L1.end L2.start
  constraint horizontal L14
  constraint vertical L15
  constraint horizontal L16
  constraint vertical L17
  constraint coincident L2.end L3.start
  constraint horizontal L18
  constraint vertical L19
  constraint horizontal L20
  constraint vertical L21
  constraint coincident L3.end L4.start
  constraint horizontal L22
  constraint vertical L23
  constraint horizontal L24
  constraint vertical L25
  constraint coincident L0.start L5.end
  constraint horizontal L26
  constraint vertical L27
  constraint horizontal L28
  constraint vertical L29
  constraint coincident L4.end L5.start
  constraint coincident L1 L30.end
  constraint perpendicular L1 L30
  constraint horizontal L32
  constraint vertical L33
  constraint horizontal L34
  constraint vertical L35
  constraint midpoint L31 L32.start
  constraint horizontal L36
  constraint vertical L37
  constraint horizontal L38
  constraint vertical L39
  constraint coincident L1 L40.end
  constraint perpendicular L1 L40
  constraint horizontal L41
  constraint vertical L42
  constraint horizontal L43
  constraint vertical L44
  constraint symmetric L30 L37.end L45.start
  constraint symmetric L30 L40.end L45.end
  constraint symmetric L30 L41.end L46.start
  constraint symmetric L30 L42.end L46.end
  constraint symmetric L30 L43.end L47.end
  constraint midpoint L52 A0.centre
  constraint midpoint L51 A1.centre
  constraint midpoint L50 A2.centre
  constraint midpoint L49 A3.centre
  constraint midpoint L55 A4.centre
  constraint midpoint L36 A5.centre
  constraint midpoint L54 A6.centre
  constraint midpoint L53 A7.centre
  measures "d291_1" distance of L0.end L6.end
  measures "d292_1" distance of L0.end L8.end
  measures "d293_1" distance of L1.end L10.end
  measures "d294_1" distance of L1.end L12.end
  measures "d295_1" distance of L2.end L14.end
  measures "d296_1" distance of L2.end L16.end
  measures "d297_1" distance of L3.end L18.end
  measures "d298_1" distance of L3.end L20.end
  measures "d299_1" distance of L0.start L22.end
  measures "d300_1" distance of L0.start L24.end
  measures "d301_1" distance of L0.start L22.end
  measures "d302_1" distance of L0.start L28.end
  measures "d303_1" distance of L32.start L32.end
  measures "d304_1" distance of L32.start L34.end
  measures "d305_1" distance of L32.start L32.end
  measures "d306_1" distance of L32.start L38.end
  measures "d307_1" distance of L40.end L41.end
  measures "d308_1" distance of L40.end L43.end
  measures "d310_1" diameter of A0
  measures "d311_1" diameter of A1
  measures "d312_1" diameter of A2
  measures "d313_1" diameter of A3
  measures "d314_1" diameter of A4
  measures "d315_1" diameter of A5
  measures "d316_1" diameter of A6
  measures "d317_1" diameter of A7
extrude "Extrude17" cut sketch "Sketch21" against normal up to surface (5 mm away) contours L55 A4 | L55 A4 | L49 A3 | L49 A3 | L32 L36 A5 | L32 L36 A5 | L50 A2 | L50 A2 | L54 A6 | L54 A6 | L51 A1 | L51 A1 | L52 A0 | L52 A0 | L53 A7 | L53 A7 bodies 2